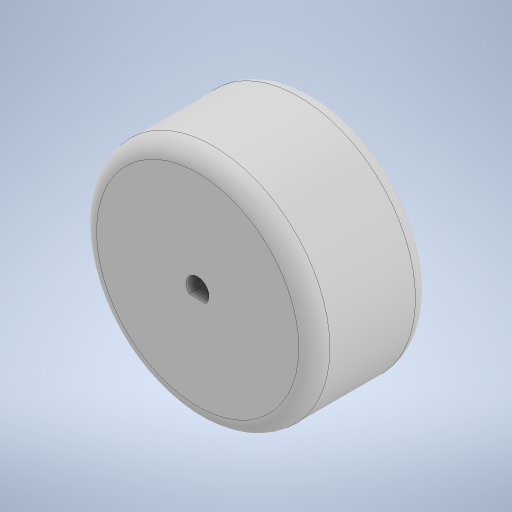
# Autodesk Inventor part: Part3
Saved by Autodesk Inventor 2024 (Build 280153000, 153)
## iProperties
Created: 2024-04-18
Part Number: Part3
Material: Generic
Document SubType Name: Modeling
Designer: Hitesh
Density: 1 g/cm^3
Appearance: Default
Author: Hitesh
Autodesk Inventor part; units mm, degrees
ref_plane "YZ Plane" through (0, 0, 0) normal (1, 0, 0) x (0, 1, 0)
ref_plane "XZ Plane" through (0, 0, 0) normal (0, 1, 0) x (-1, 0, 0)
ref_plane "XY Plane" through (0, 0, 0) normal (0, 0, 1) x (1, 0, 0)
sketch "Sketch1" plane through (0, 0, 0) normal (0, 0, 1) x (1, 0, 0)
  circle A0 centre (0, 0) radius 15
  arc A1 (1.0844, -0.985) -> (-1.0844, -0.985) centre (0, 0) ccw
  line L0 (1.0844, -0.985) -> (-1.0844, -0.985)
  dimension "d0" = 30
  dimension "d1" = 2.93
  dimension "d2" = 2.45
  constraints: 2 centre point, 2 coincident, 2 end point, 2 point on circle, 1 horizontal
  measures "d0" diameter of A0
  measures "d1" diameter of A1
extrude "Extrusion1" add sketch "Sketch1" along normal blind 15
fillet "Fillet1" radius 2 2 edges at (-15, 0, 15) (-15, 0, 0)
body "Solid1"
